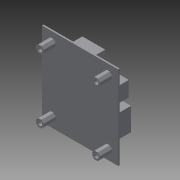
# Autodesk Inventor part: carte_puissance
Saved by Autodesk Inventor 2014 SP1 (Build 180222100, 222)
## iProperties
Created: 2015-02-02
Part Number: carte_puissance
Material: Générique
Document SubType Name: Modeling
Designer: astralien3000
Density: 1 g/cm^3
Appearance: Par défaut
Author: astralien3000
Autodesk Inventor part; units mm, degrees
ref_plane "YZ Plane" through (0, 0, 0) normal (1, 0, 0) x (0, 1, 0)
ref_plane "XZ Plane" through (0, 0, 0) normal (0, 1, 0) x (-1, 0, 0)
ref_plane "XY Plane" through (0, 0, 0) normal (0, 0, 1) x (1, 0, 0)
sketch "Esquisse1" plane through (0, 0, 0) normal (0, 1, 0) x (-1, 0, 0)
  line L0 (-25, 27.5) -> (25, 27.5)
  line L1 (25, 27.5) -> (25, -27.5)
  line L2 (25, -27.5) -> (-25, -27.5)
  line L3 (-25, -27.5) -> (-25, 27.5)
  point P0 (0, 0)
  dimension "d0" = 55
  dimension "d1" = 50
  dimension "d2" = 25
  dimension "d3" = 27.5
  constraints: 8 end point, 2 parallel, 1 horizontal, 1 perpendicular
  measures "d0" distance of L2.end L0.start
  measures "d1" distance of L0.start L0.end
  measures "d2" distance from line of L1 point (0, 0)
  measures "d3" distance from line of L0 point (0, 0)
extrude "Extrusion1" add sketch "Esquisse1" along normal blind 1
sketch "Esquisse2" plane through (0, 1, 0) normal (0, 1, 0) x (1, 0, 0)
  line L0 (25, 27.5) -> (-25, 27.5) projected
  line L1 (-12.5, 25) -> (12.5, 25)
  line L2 (12.5, 25) -> (12.5, 10)
  line L3 (12.5, 10) -> (-12.5, 10)
  line L4 (-12.5, 10) -> (-12.5, 25)
  point P0 (0, 0)
  dimension "d6" = 15
  dimension "d7" = 25
  dimension "d8" = 12.5
  dimension "d9" = 2.5
  constraints: 8 end point, 2 parallel, 1 horizontal, 1 perpendicular
  measures "d6" distance of L3.end L1.start
  measures "d7" distance of L2.end L3.end
  measures "d8" distance from line of point (0, 0) L2
  measures "d9" distance between parallel lines of L0 L1
extrude "Extrusion2" add sketch "Esquisse2" along normal blind 20
sketch "Esquisse3" plane through (0, 1, 0) normal (0, 1, 0) x (1, 0, 0)
  line L0 (-25, -27.5) -> (25, -27.5) projected
  line L1 (25, -27.5) -> (25, 27.5) projected
  line L2 (-25, 27.5) -> (-25, -27.5) projected
  line L3 (-23, -6) -> (-15, -6)
  line L4 (-15, -6) -> (-15, -16)
  line L5 (-15, -16) -> (-23, -16)
  line L6 (-23, -16) -> (-23, -6)
  line L7 (15, -6) -> (23, -6)
  line L8 (23, -6) -> (23, -16)
  line L9 (23, -16) -> (15, -16)
  line L10 (15, -16) -> (15, -6)
  line L11 (-7.5, -17.5) -> (7.5, -17.5)
  line L12 (7.5, -17.5) -> (7.5, -25.5)
  line L13 (7.5, -25.5) -> (-7.5, -25.5)
  line L14 (-7.5, -25.5) -> (-7.5, -17.5)
  line L15 (-5, -9.5) -> (5, -9.5)
  line L16 (5, -9.5) -> (5, -14.5)
  line L17 (5, -14.5) -> (-5, -14.5)
  line L18 (-5, -14.5) -> (-5, -9.5)
  point P0 (0, 0)
  dimension "d12" = 10
  dimension "d13" = 10
  dimension "d14" = 10
  dimension "d15" = 8
  dimension "d16" = 8
  dimension "d17" = 15
  dimension "d18" = 8
  dimension "d19" = 5
  dimension "d20" = 5
  dimension "d21" = 2
  dimension "d22" = 2
  dimension "d23" = 2
  dimension "d24" = 7.5
  dimension "d25" = 6
  dimension "d26" = 3
  constraints: 32 end point, 8 parallel, 4 horizontal, 4 perpendicular, 1 collinear
  measures "d12" distance of L15.start L15.end
  measures "d13" distance of L7.end L8.end
  measures "d14" distance of L5.end L3.start
  measures "d15" distance of L3.start L3.end
  measures "d16" distance of L7.start L7.end
  measures "d17" distance of L12.end L13.end
  measures "d18" distance of L11.end L12.end
  measures "d19" distance of L15.end L16.end
  measures "d20" distance from line of point (0, 0) L16
  measures "d21" distance between parallel lines of L0 L13
  measures "d22" distance between parallel lines of L1 L8
  measures "d23" distance between parallel lines of L2 L6
  measures "d24" distance from line of point (0, 0) L12
  measures "d25" distance from line of point (0, 0) L3
  measures "d26" distance between parallel lines of L11 L17
extrude "Extrusion3" add sketch "Esquisse3" along normal blind 8
sketch "Esquisse4" plane through (0, 0, 0) normal (0, -1, 0) x (1, 0, 0)
  line L0 (25, 27.5) -> (-25, 27.5) projected
  line L1 (-25, 27.5) -> (-25, -27.5) projected
  line L2 (-19.5355, 23.5) -> (-17.4645, 23.5)
  line L3 (-17.4645, 23.5) -> (-17.4645, 18.5) construction
  line L4 (-17.4645, 18.5) -> (-19.5355, 18.5)
  line L5 (-19.5355, 18.5) -> (-19.5355, 23.5) construction
  line L6 (-21, 22.0355) -> (-16, 22.0355) construction
  line L7 (-16, 22.0355) -> (-16, 19.9645)
  line L8 (-16, 19.9645) -> (-21, 19.9645) construction
  line L9 (-21, 19.9645) -> (-21, 22.0355)
  line L10 (-21, 22.0355) -> (-19.5355, 23.5)
  line L11 (-17.4645, 23.5) -> (-16, 22.0355)
  line L12 (-16, 19.9645) -> (-17.4645, 18.5)
  line L13 (-19.5355, 18.5) -> (-21, 19.9645)
  line L14 (-19.5355, 22.0355) -> (-17.4645, 19.9645) construction
  line L15 (-17.4645, 22.0355) -> (-19.5355, 19.9645) construction
  circle A0 centre (-18.5, 21) radius 1.5
  line L16 (0, 0) -> (0, 27.5) construction
  line L17 (0, 0) -> (-25, 0) construction
  line L18 (19.5355, 23.5) -> (17.4645, 23.5)
  line L19 (17.4645, 23.5) -> (17.4645, 18.5) construction
  line L20 (17.4645, 18.5) -> (19.5355, 18.5)
  line L21 (19.5355, 18.5) -> (19.5355, 23.5) construction
  line L22 (21, 22.0355) -> (16, 22.0355) construction
  line L23 (16, 22.0355) -> (16, 19.9645)
  line L24 (16, 19.9645) -> (21, 19.9645) construction
  line L25 (21, 19.9645) -> (21, 22.0355)
  line L26 (21, 22.0355) -> (19.5355, 23.5)
  line L27 (17.4645, 23.5) -> (16, 22.0355)
  line L28 (16, 19.9645) -> (17.4645, 18.5)
  line L29 (19.5355, 18.5) -> (21, 19.9645)
  line L30 (19.5355, 22.0355) -> (17.4645, 19.9645) construction
  line L31 (17.4645, 22.0355) -> (19.5355, 19.9645) construction
  circle A1 centre (18.5, 21) radius 1.5
  line L32 (-19.5355, -23.5) -> (-17.4645, -23.5)
  line L33 (-17.4645, -23.5) -> (-17.4645, -18.5) construction
  line L34 (-17.4645, -18.5) -> (-19.5355, -18.5)
  line L35 (-19.5355, -18.5) -> (-19.5355, -23.5) construction
  line L36 (-21, -22.0355) -> (-16, -22.0355) construction
  line L37 (-16, -22.0355) -> (-16, -19.9645)
  line L38 (-16, -19.9645) -> (-21, -19.9645) construction
  line L39 (-21, -19.9645) -> (-21, -22.0355)
  line L40 (-21, -22.0355) -> (-19.5355, -23.5)
  line L41 (-17.4645, -23.5) -> (-16, -22.0355)
  line L42 (-16, -19.9645) -> (-17.4645, -18.5)
  line L43 (-19.5355, -18.5) -> (-21, -19.9645)
  line L44 (-19.5355, -22.0355) -> (-17.4645, -19.9645) construction
  line L45 (-17.4645, -22.0355) -> (-19.5355, -19.9645) construction
  circle A2 centre (-18.5, -21) radius 1.5
  line L46 (16, -19.9645) -> (17.4645, -18.5)
  line L47 (17.4645, -18.5) -> (19.5355, -18.5)
  line L48 (16, -22.0355) -> (16, -19.9645)
  line L49 (16, -19.9645) -> (21, -19.9645) construction
  line L50 (19.5355, -18.5) -> (21, -19.9645)
  line L51 (17.4645, -23.5) -> (17.4645, -18.5) construction
  line L52 (17.4645, -23.5) -> (16, -22.0355)
  line L53 (19.5355, -22.0355) -> (17.4645, -19.9645) construction
  line L54 (17.4645, -22.0355) -> (19.5355, -19.9645) construction
  circle A3 centre (18.5, -21) radius 1.5
  line L55 (21, -22.0355) -> (16, -22.0355) construction
  line L56 (21, -19.9645) -> (21, -22.0355)
  line L57 (19.5355, -18.5) -> (19.5355, -23.5) construction
  line L58 (19.5355, -23.5) -> (17.4645, -23.5)
  line L59 (21, -22.0355) -> (19.5355, -23.5)
  dimension "d29" = 5
  dimension "d30" = 5
  dimension "d31" = 4
  dimension "d32" = 4
  dimension "d35" = 3
  constraints: 116 end point, 39 symmetric about line, 32 point on line, 5 perpendicular, 4 centre point, 4 parallel, 3 midpoint, 2 horizontal, 1 equal length, 3 other
  measures "d29" distance of L6.start L6.end
  measures "d30" distance of L4.end L2.start
  measures "d31" distance between parallel lines of L1 L9
  measures "d32" distance between parallel lines of L0 L2
  measures "d35" diameter of A0
extrude "Extrusion4" add sketch "Esquisse4" along normal blind 8
equation "\"d2\" = 0.5 * d1"
equation "\"d3\" = 0.5 * d0"
equation "\"d8\" = 0.5 * d7"
equation "\"d14\" = d13"
equation "\"d16\" = d15"
equation "\"d20\" = 0.5 * d12"
equation "\"d22\" = d21"
equation "\"d23\" = d21"
equation "\"d24\" = 0.5 * d17"
equation "\"d30\" = d29"
